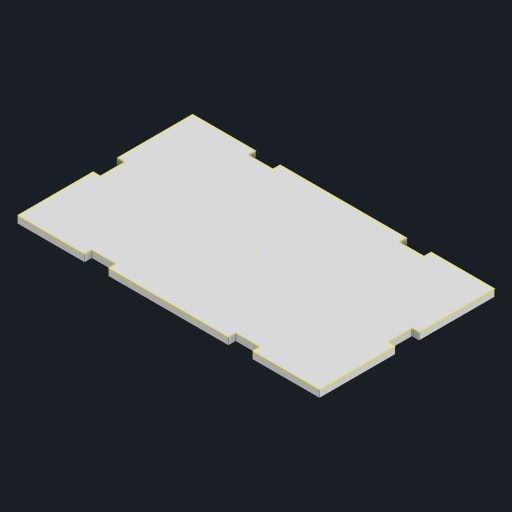
# Autodesk Inventor part: top
Saved by Autodesk Inventor 2023 (Build 270158000, 158)
## iProperties
Created: 2024-07-21
Part Number: top
Material: Generic
Document SubType Name: Modeling
Designer: Orsted
Density: 1 g/cm^3
Appearance: Default
Author: Orsted
Autodesk Inventor part; units mm, degrees
ref_plane "YZ Plane" through (0, 0, 0) normal (1, 0, 0) x (0, 1, 0)
ref_plane "XZ Plane" through (0, 0, 0) normal (0, 1, 0) x (-1, 0, 0)
ref_plane "XY Plane" through (0, 0, 0) normal (0, 0, 1) x (1, 0, 0)
sketch "Sketch1" plane through (0, 0, 0) normal (0, 1, 0) x (-1, 0, 0)
  line L0 (-63, -36.5) -> (63, -36.5)
  line L1 (63, -36.5) -> (63, 36.5)
  line L2 (63, 36.5) -> (-63, 36.5)
  line L3 (-63, 36.5) -> (-63, -36.5)
  line L4 (-63, -36.5) -> (63, 36.5) construction
  line L5 (63, -36.5) -> (-63, 36.5) construction
  point P0 (0, 0)
  dimension "d0" = 126
  dimension "d1" = 73
  constraints: 12 end point, 2 midpoint, 2 parallel, 1 horizontal, 1 perpendicular
  measures "d0" distance of L2.end L1.end
  measures "d1" distance of L1.end L0.end
extrude "Extrusion1" add sketch "Sketch1" along normal blind 3
sketch "Sketch3" plane through (0, 3, 0) normal (0, 1, 0) x (1, 0, 0)
  line L0 (-25, -33.5) -> (25, -33.5)
  line L1 (-35, -33.5) -> (-25, -33.5)
  line L2 (-60, -33.5) -> (-35, -33.5)
  line L3 (-60, -5) -> (-60, -36.5)
  line L4 (-60, 5) -> (-60, -5)
  line L5 (-60, 36.5) -> (-60, 5)
  line L6 (-36.5, 33.5) -> (-60, 33.5)
  line L7 (-26.5, 33.5) -> (-36.5, 33.5)
  line L8 (26.5, 33.5) -> (-26.5, 33.5)
  line L9 (36.5, 33.5) -> (26.5, 33.5)
  line L10 (60, 33.5) -> (36.5, 33.5)
  line L11 (60, 5) -> (60, 36.5)
  line L12 (60, -5) -> (60, 5)
  line L13 (60, -36.5) -> (60, -5)
  line L14 (35, -33.5) -> (60, -33.5)
  line L15 (25, -33.5) -> (35, -33.5)
  line L16 (-35, -36.5) -> (-35, -33.5)
  line L17 (-25, -36.5) -> (-25, -33.5)
  line L18 (25, -36.5) -> (25, -33.5)
  line L19 (35, -36.5) -> (35, -33.5)
  line L20 (-36.5, 36.5) -> (-36.5, 33.5)
  line L21 (-26.5, 36.5) -> (-26.5, 33.5)
  line L22 (26.5, 36.5) -> (26.5, 33.5)
  line L23 (36.5, 36.5) -> (36.5, 33.5)
  line L24 (-60, 5) -> (-63, 5)
  line L25 (-63, -5) -> (-60, -5)
  line L26 (63, 5) -> (60, 5)
  line L27 (60, -5) -> (63, -5)
  line L28 (63, -36.5) -> (63, 36.5) projected
  line L29 (63, 36.5) -> (-63, 36.5) projected
  line L30 (-63, 36.5) -> (-63, -36.5) projected
  line L31 (-63, -36.5) -> (63, -36.5) projected
  point P0 (0, 0)
  constraints: 56 end point, 14 horizontal, 14 vertical, 32 other
extrude "Extrusion3" cut sketch "Sketch3" against normal through all contours L17 L31 L16 L1 | L15 L19 L31 L18 | L25 L30 L24 L4 | L12 L26 L28 L27 | L20 L29 L21 L7 | L9 L22 L29 L23
sketch "Sketch4" plane through (0, 3, 0) normal (0, 1, 0) x (1, 0, 0)
  line L0 (-63, -5) -> (-60, -5) projected
  line L1 (-60, -5) -> (-60, 5) projected
  line L2 (-60, 5) -> (-63, 5) projected
  line L3 (-63, 5) -> (-63, 36.5) projected
  line L4 (-63, 36.5) -> (-36.5, 36.5) projected
  line L5 (-36.5, 36.5) -> (-36.5, 33.5) projected
  line L6 (-36.5, 33.5) -> (-26.5, 33.5) projected
  line L7 (-26.5, 33.5) -> (-26.5, 36.5) projected
  line L8 (-26.5, 36.5) -> (26.5, 36.5) projected
  line L9 (26.5, 36.5) -> (26.5, 33.5) projected
  line L10 (26.5, 33.5) -> (36.5, 33.5) projected
  line L11 (36.5, 33.5) -> (36.5, 36.5) projected
  line L12 (36.5, 36.5) -> (63, 36.5) projected
  line L13 (63, 36.5) -> (63, 5) projected
  line L14 (63, 5) -> (60, 5) projected
  line L15 (60, 5) -> (60, -5) projected
  line L16 (60, -5) -> (63, -5) projected
  line L17 (63, -5) -> (63, -36.5) projected
  line L18 (63, -36.5) -> (35, -36.5) projected
  line L19 (35, -36.5) -> (35, -33.5) projected
  line L20 (35, -33.5) -> (25, -33.5) projected
  line L21 (25, -33.5) -> (25, -36.5) projected
  line L22 (25, -36.5) -> (-25, -36.5) projected
  line L23 (-25, -36.5) -> (-25, -33.5) projected
  line L24 (-25, -33.5) -> (-35, -33.5) projected
  line L25 (-35, -33.5) -> (-35, -36.5) projected
  line L26 (-35, -36.5) -> (-63, -36.5) projected
  line L27 (-63, -36.5) -> (-63, -5) projected
  point P0 (0, 0)
body "Solid1"
